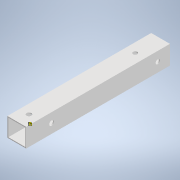
# Autodesk Inventor part: 4_barra
Saved by Autodesk Inventor 2020 (Build 240168000, 168)
## iProperties
Created: 2019-10-11
Part Number: 4_barra
Material: Generico
Document SubType Name: Modeling
Designer: socci
Density: 1 g/cm^3
Appearance: Default
Author: socci
Autodesk Inventor part; units mm, degrees
ref_plane "YZ Plane" through (0, 0, 0) normal (1, 0, 0) x (0, 1, 0)
ref_plane "XZ Plane" through (0, 0, 0) normal (0, 1, 0) x (-1, 0, 0)
ref_plane "XY Plane" through (0, 0, 0) normal (0, 0, 1) x (1, 0, 0)
sketch "Schizzo1" plane through (0, 0, 0) normal (0, 0, 1) x (1, 0, 0)
  line L0 (10, -10) -> (-10, -10)
  line L1 (-10, -10) -> (-10, 10)
  line L2 (-10, 10) -> (10, 10)
  line L3 (10, 10) -> (10, -10)
  line L4 (9, 9) -> (-9, 9)
  line L5 (-9, 9) -> (-9, -9)
  line L6 (-9, -9) -> (9, -9)
  line L7 (9, -9) -> (9, 9)
  point P0 (0, 0)
  point P1 (0, 0)
  dimension "d0" = 20
  dimension "d1" = 1
  constraints: 16 end point, 1 coincident, 12 other
  measures "d0" distance of L1.end L2.end
  measures "d1" distance between parallel lines of L2 L4
extrude "Estrusione1" add sketch "Schizzo1" against normal blind 153
sketch "Schizzo2" plane through (-10, 10, 0) normal (0, 1, 0) x (1, 0, 0)
  circle A0 centre (10, 13) radius 2.5 projected
  point P0 (10, 0)
hole "Foro1" at (0, 10, -13) direction (0, -1, 0) diameter 5 end through all
sketch "Schizzo3" plane through (10, -10, 0) normal (1, 0, 0) x (0, 0, -1)
  circle A0 centre (27, 10) radius 2.5 projected
  point P0 (0, 10)
hole "Foro2" at (10, 0, -27) direction (-1, 0, 0) diameter 5 end through all
sketch "Schizzo6" plane through (10, -10, 0) normal (1, 0, 0) x (0, 0, -1)
  circle A0 centre (140, 10) radius 2.5 projected
  circle A1 centre (140, 10) radius 2.5
  point P0 (0, 10)
  constraints: 1 centre point, 1 coincident, 1 concentric
hole "Foro5" at (10, 0, -140) direction (-1, 0, 0) diameter 4.5 end through all clearance for "Vite a testa piana" size "M4" standard "ANSI - Profilo M Metrico"
sketch "Schizzo7" plane through (-10, 10, 0) normal (0, 1, 0) x (1, 0, 0)
  circle A0 centre (10, 13) radius 2.5 projected
  line L0 (20, 0) -> (0, 0) projected
  line L1 (20, 0) -> (20, 153) projected
  line L2 (0, 153) -> (20, 153) projected
  line L3 (0, 0) -> (0, 153) projected
  circle A1 centre (10, 126) radius 2.5 projected
  circle A2 centre (10, 126) radius 2.5
  point P0 (10, 0)
  constraints: 1 centre point, 1 coincident, 1 concentric
hole "Foro6" at (0, 10, -126) direction (0, -1, 0) diameter 4.5 end through all clearance for "Vite a testa piana" size "M4" standard "ANSI - Profilo M Metrico"
